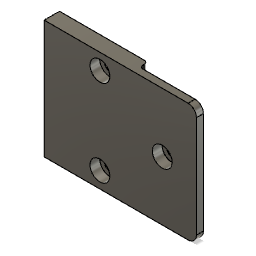
EBike Battery Mount Lid (Autodesk Fusion 360 design; units mm, degrees)
Autodesk Fusion 360 part; units mm, degrees
sketch "Sketch1" plane through (0, 0, 0) normal (0, 0, 1) x (1, 0, 0)
  line L0 (27.32, 21.5) -> (-27.32, 21.5) construction
  line L1 (-27.32, 21.5) -> (-27.32, -21.5) construction
  line L2 (-27.32, -21.5) -> (27.32, -21.5) construction
  line L3 (27.32, -21.5) -> (27.32, 21.5) construction
  line L4 (27.32, 21.5) -> (-27.32, -21.5) construction
  line L5 (-27.32, 21.5) -> (27.32, -21.5) construction
  line L6 (-27.32, 21.246) -> (27.32, 21.246)
  line L7 (27.32, 21.246) -> (27.32, -21.246)
  line L8 (-27.32, 21.246) -> (-27.32, -21.246)
  line L9 (-27.32, 0) -> (0, 0) construction
  line L10 (-27.32, -21.246) -> (27.32, -21.246)
  dimension "d1" = 54.64
  dimension "d2" = 43
  dimension "d19" = 0.254
  constraint horizontal L0
  constraint perpendicular L0 L1
  constraint parallel L0 L2
  constraint parallel L1 L3
  constraint coincident L4 L9.end
  constraint coincident L5 L9.end
  constraint coincident L9.end origin
  constraint coincident L1 L6.start
  constraint coincident L3 L6.end
  constraint perpendicular L3 L6
  constraint coincident L3 L7.end
  constraint midpoint L8 L9.start
  constraint coincident L1 L8.end
  constraint parallel L1 L8
  constraint horizontal L9
  constraint horizontal L10
  measures "d1" distance of L0.start L0.end
  measures "d2" distance of L0.end L1.end
  measures "d19" distance of L0 L6
extrude "Extrude1" add sketch "Sketch1" along normal blind 2.513
sketch "Sketch2" plane through (0, 0, 0) normal (0, 0, -1) x (-1, 0, 0)
  line L0 (27.32, 21.246) -> (-4.355, 21.246)
  line L1 (-4.355, 21.246) -> (-4.355, -21.246)
  line L2 (-4.355, -21.246) -> (27.32, -21.246)
  line L3 (27.32, -21.246) -> (27.32, 21.246)
  line L4 (27.32, -21.246) -> (27.32, 21.246)
  line L5 (27.32, 21.246) -> (-27.32, 21.246)
  line L6 (-27.32, 21.246) -> (-27.32, -21.246)
  line L7 (-27.32, -21.246) -> (27.32, -21.246)
  dimension "d5" = 31.675
  constraint horizontal L0
  constraint vertical L1
  constraint horizontal L2
  constraint vertical L3
  constraint coincident L0.end L5
  constraint coincident L1.end L7
  constraint coincident L0.start L3.end
  measures "d5" distance of L0.end L0.start
extrude "Extrude2" add sketch "Sketch2" along normal blind 2.987 contours L0 L1 L2 L3 L4 L5 L7
fillet "Fillet1" radius 3 2 edges at (27.32, 21.246, 1.2565) (27.32, -21.246, 1.2565)
sketch "Sketch5" plane through (0, 0, 0) normal (0, 0, -1) x (-1, 0, 0)
  line L0 (-4.355, 21.246) -> (-24.32, 21.246)
  arc A0 (-24.32, 21.246) -> (-27.32, 18.246) centre (-24.32, 18.246) ccw
  line L1 (-27.32, 18.246) -> (-27.32, -18.246)
  arc A1 (-27.32, -18.246) -> (-24.32, -21.246) centre (-24.32, -18.246) ccw
  line L2 (-24.32, -21.246) -> (-4.355, -21.246)
  line L3 (-20.54, 7) -> (-9.54, 7) construction
  line L4 (-9.54, 7) -> (-9.54, -7) construction
  line L5 (-9.54, -7) -> (-20.54, -7) construction
  line L6 (-20.54, -7) -> (-20.54, 7) construction
  line L7 (-27.32, 0) -> (-20.54, 0) construction
  line L8 (-9.794, -6.746) -> (-20.286, -6.746)
  line L9 (-20.286, -6.746) -> (-20.286, 6.746)
  line L10 (-20.286, 6.746) -> (-9.794, 6.746)
  line L11 (-9.794, 6.746) -> (-9.794, -6.746)
  line L12 (-4.355, -21.246) -> (-4.355, 21.246)
  dimension "d34" = 6.78
  dimension "d35" = 11
  dimension "d38" = 0.254
  dimension "d46" = 14
  constraint horizontal L3
  constraint vertical L4
  constraint horizontal L5
  constraint vertical L6
  constraint midpoint L1 L7.start
  constraint midpoint L6 L7.end
  constraint horizontal L7
  measures "d34" distance of L1 L6
  measures "d35" distance of L3.start L3.end
  measures "d46" distance of L3.end L4.end
extrude "Extrude4" add sketch "Sketch5" along normal blind 2.9986 contours L8 L9 L10 L11
sketch "Sketch3" plane through (0, 0, 2.513) normal (0, 0, 1) x (1, 0, 0)
  line L0 (27.32, 21.5) -> (-27.32, 21.5) construction
  line L1 (-27.32, -21.5) -> (27.32, -21.5) construction
  line L2 (-27.32, 21.246) -> (-27.32, -21.246) construction
  line L3 (27.32, 21.246) -> (27.32, -21.246) construction
  line L4 (-27.32, 0) -> (0, 0) construction
  line L5 (0, 0) -> (27.32, 0) construction
  line L6 (15.04, 0) -> (15.04, 6.746) construction
  line L7 (9.794, 6.746) -> (20.286, 6.746) construction
  point P0 (-7.32, -15.5)
  point P1 (-7.32, 15.5)
  point P2 (15.04, 0)
  dimension "d25" = 6
  dimension "d28" = 20
  constraint midpoint L2 L4.start
  constraint coincident L4.end L5.start
  constraint symmetric P0 L4 P1
  constraint midpoint L3 L5.end
  constraint coincident L5 P2
  constraint coincident P2 L6.start
  constraint perpendicular L5 L6
  constraint midpoint L6.end L7
  measures "d25" distance of L0 P1
  measures "d28" distance of L2 P1
hole "Hole1" at (-7.32, 15.5, 2.513) at (-7.32, -15.5, 2.513) at (15.04, 0, 2.513) direction (0, 0, -1) diameter 3.81 depth 39.751 tip angle 118 counterbore diameter 7.1374 counterbore depth 3.5052
fillet "Fillet2" radius 1.27 2 edges at (4.355, 0, 0) (4.355, 0, -2.987)
sketch "Sketch4" plane through (-27.32, 0, 0) normal (-1, 0, 0) x (0, 0, 1)
  line L0 (-2.987, -21.246) -> (2.513, -21.246)
  line L1 (2.513, -21.246) -> (2.513, 21.246)
  line L2 (2.513, 21.246) -> (-2.987, 21.246)
  line L3 (-2.987, 21.246) -> (-2.987, -21.246)
  line L4 (-2.3774, -4.0546) -> (-2.3774, 4.0546) construction
  line L5 (0, 0) -> (-2.3774, 0) construction
  line L6 (-2.987, 9.4361) -> (0.0102, 9.4361)
  line L7 (0.0102, 9.4361) -> (0.0102, -9.4361)
  line L8 (0.0102, -9.4361) -> (-2.987, -9.4361)
  line L9 (-2.987, -9.4361) -> (-2.987, 9.4361)
  line L10 (0, 0) -> (0.0102, 0) construction
  dimension "d30" = 2.3876
  dimension "d31" = 18.8722
  dimension "d41" = 0.6096
  constraint vertical L4
  constraint coincident L5.start L10.start
  constraint midpoint L4 L5.end
  constraint horizontal L5
  constraint horizontal L6
  constraint vertical L7
  constraint horizontal L8
  constraint vertical L9
  constraint coincident L3 L6.start
  constraint midpoint L7 L10.end
  constraint horizontal L10
  measures "d30" distance of L4 L7
  measures "d31" distance of L6.end L7.end
  measures "d41" distance of L4 L9
extrude "Extrude3" cut sketch "Sketch4" against normal blind 9.2964 contours L3 L6 L7 L8 L9
fillet "Fillet3" radius 1.5 4 edges at (20.286, 6.746, -1.4993) (9.794, 6.746, -1.4993) (20.286, -6.746, -1.4993) (9.794, -6.746, -1.4993)
sketch "Sketch6" plane through (0, 0, -2.987) normal (0, 0, -1) x (-1, 0, 0)
  circle A0 centre (7.32, 15.5) radius 1.905
  circle A1 centre (7.32, -15.5) radius 1.905
  line L0 (27.32, -9.4361) -> (18.0236, -9.4361)
  line L1 (18.0236, -9.4361) -> (18.0236, 9.4361)
  line L2 (18.0236, 9.4361) -> (27.32, 9.4361)
  line L3 (27.32, 9.4361) -> (27.32, 21.246)
  line L4 (27.32, 21.246) -> (-3.085, 21.246)
  line L5 (-3.085, 21.246) -> (-3.085, -21.246)
  line L6 (-3.085, -21.246) -> (27.32, -21.246)
  line L7 (27.32, -21.246) -> (27.32, -9.4361)
  line L8 (18.0236, 9.4361) -> (1.0236, 9.4361)
  line L9 (1.0236, 9.4361) -> (1.0236, -9.4361)
  line L10 (1.0236, -9.4361) -> (18.0236, -9.4361)
  line L11 (18.0236, -9.4361) -> (18.0236, 9.4361)
  line L12 (0, 0) -> (1.0236, 0) construction
  dimension "d43" = 17
  constraint horizontal L8
  constraint vertical L9
  constraint horizontal L10
  constraint vertical L11
  constraint coincident L1 L2.start
  constraint coincident L12.start origin
  constraint midpoint L9 L12.end
  constraint horizontal L12
  constraint collinear L2 L8
  measures "d43" distance of L1.end L8.end
extrude "Extrude5" cut sketch "Sketch6" against normal blind 2.2 contours L1 L8 L9 L10 L11
equation "d6 = 1.487 mm + 1.5 mm"
equation "d36 = 0.059 in + 1.5 mm"
